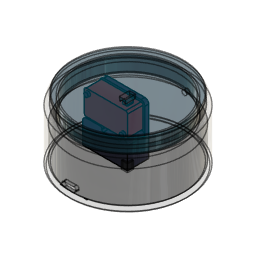
feeder (Autodesk Fusion 360 design; units mm, degrees)
part number: 2025-06-02-16-29-52-871
Autodesk Fusion 360 part; units mm, degrees
note: some values were not read from the file. Chosen so that the rebuilt part matches the saved one: which bodies a step acts on. Set by a fixed rule: which sketch regions a step uses.
sketch "Esquisse1" plane through (0, 0, 0) normal (0, 0, 1) x (1, 0, 0)
  circle A0 centre (0, 0) radius 35.5
  dimension "d1" = 71
  constraint coincident A0.centre origin
  measures "d1" diameter of A0
extrude "Extrusion1" add sketch "Esquisse1" along normal blind 2 makes body 1
sketch "Esquisse3" plane through (0, 0, 0) normal (0, 1, 0) x (1, 0, 0)
  line L0 (38.5, -1) -> (38.5, 38)
  line L1 (37.5, 39) -> (0, 39)
  line L2 (0, 39) -> (0, 37)
  line L3 (0, 37) -> (33, 37)
  line L4 (33, 37) -> (35.5, 37)
  line L5 (36.5, 36) -> (36.5, 8)
  arc A0 (36.5, 36) -> (35.5, 37) centre (35.5, 36) ccw
  arc A1 (38.5, 38) -> (37.5, 39) centre (37.5, 38) ccw
  line L6 (36, -1) -> (38.5, -1)
  line L7 (36, -1) -> (36, 4.6069)
  line L8 (36, 4.6069) -> (33, 4.6069)
  line L9 (33, 4.6069) -> (33, 12.1069)
  line L10 (33, 12.1069) -> (36.5, 15.6069)
  line L11 (33, 12.1069) -> (37.9497, 12.1069) construction
  point P0 (36.5, 37)
  dimension "d19" = 2
  dimension "d20" = 3.5
  dimension "d21" = 1
  dimension "d120" = 7.5
  dimension "d121" = 45
  constraint perpendicular L0 L1
  constraint perpendicular L1 L2
  constraint perpendicular L0 L4
  constraint perpendicular L4 L5
  constraint coincident P0 L4
  constraint coincident P0 L5
  constraint tangent L4 A0
  constraint tangent L5 A0
  constraint tangent L1 A1
  constraint tangent L0 A1
  constraint equal A0 A1
  constraint perpendicular L0 L6
  constraint horizontal L6
  constraint perpendicular L7 L8
  constraint perpendicular L8 L9
  constraint horizontal L11
  constraint coincident L5 L10.end
  measures "d19" distance of L1.end L2.end
  measures "d20" distance of L3.end P0
  measures "d21" radius of A0
  measures "d120" distance of L8.end L9.end
  measures "d121" angle of L10 L11
revolve "Révolution2" add sketch "Esquisse3" angle 360 about axis through (0, 0, 1.75) along (0, 0, 1) separate body makes body 2
sketch "Esquisse5" plane through (0, 0, 0) normal (0, 0, 1) x (1, 0, 0)
  line L0 (75, 0) -> (103, 0)
  line L1 (103, 0) -> (103, -16)
  line L2 (103, -16) -> (75, -16)
  line L3 (75, -16) -> (75, 0)
  dimension "d23" = 28
  dimension "d24" = 16
  constraint horizontal L0
  constraint vertical L1
  constraint horizontal L2
  constraint vertical L3
  measures "d23" distance of L0.start L0.end
  measures "d24" distance of L0.start L2.end
extrude "Extrusion4" add sketch "Esquisse5" along normal blind 10 separate body makes body 3
sketch "Esquisse6" plane through (0, 0, 0) normal (0, 1, 0) x (-1, 0, 0)
  line L0 (-103, 0) -> (-75, 0)
  line L1 (-75, 0) -> (-75, 10)
  line L2 (-75, 10) -> (-103, 10)
  line L3 (-103, 10) -> (-103, 0)
  line L4 (-89, 0) -> (-89, 10)
  line L5 (-75, 5) -> (-103, 5)
  line L6 (-103, 5) -> (-99.8, 5)
  line L7 (-99.8, 5) -> (-96.8, 5)
  line L8 (-98.3, 5) -> (-98.3, 3)
  line L9 (-96.8, 3) -> (-99.8, 3)
  line L10 (-99.8, 3) -> (-99.8, 7)
  line L11 (-99.8, 7) -> (-96.8, 7)
  line L12 (-96.8, 7) -> (-96.8, 3)
  dimension "d27" = 3.2
  dimension "d28" = 3
  dimension "d29" = 2
  dimension "d30" = 3
  dimension "d31" = 4
  constraint midpoint L0 L4.start
  constraint midpoint L2 L4.end
  constraint midpoint L1 L5.start
  constraint midpoint L3 L5.end
  constraint perpendicular L3 L6
  constraint perpendicular L3 L7
  constraint midpoint L7 L8.start
  constraint perpendicular L5 L8
  constraint horizontal L9
  constraint vertical L10
  constraint horizontal L11
  constraint vertical L12
  measures "d27" distance of L5.end L6.end
  measures "d28" distance of L6.end L7.end
  measures "d29" distance of L8.start L8.end
  measures "d30" distance of L9.start L9.end
  measures "d31" distance of L9.start L11.end
extrude "Extrusion5" add sketch "Esquisse6" along normal blind 2.3 contours L5 L7 L10 L11 L12 | L5 L7 L8 L9 L10 | L5 L7 L8 L9 L12 bodies 3
fillet "Congé1" radius 1.5 2 edges at (99.8, 2.3, 5) (96.8, 2.3, 5) on bodies 3
fillet "Congé2" radius 1.25 4 edges at (103, 0, 5) (75, 0, 5) (103, -16, 5) (75, -16, 5) on bodies 3
sketch "Esquisse7" plane through (0, 0, 10) normal (0, 0, 1) x (-1, 0, 0)
  arc A0 (-75, 14.75) -> (-76.25, 16) centre (-76.25, 14.75) ccw
  line L0 (-76.25, 16) -> (-101.75, 16)
  arc A1 (-101.75, 16) -> (-103, 14.75) centre (-101.75, 14.75) ccw
  line L1 (-103, 14.75) -> (-103, 1.25)
  arc A2 (-103, 1.25) -> (-101.75, 0) centre (-101.75, 1.25) ccw
  line L2 (-101.75, 0) -> (-76.25, 0)
  arc A3 (-76.25, 0) -> (-75, 1.25) centre (-76.25, 1.25) ccw
  line L3 (-75, 1.25) -> (-75, 14.75)
  line L4 (-77.5, 0) -> (-77.5, 2.5)
  line L5 (-75, 2.5) -> (-77.5, 2.5)
  line L6 (-100.5, 16) -> (-100.5, 13.5)
  line L7 (-103, 13.5) -> (-100.5, 13.5)
  circle A4 centre (-77.5, 2.5) radius 1.5
  circle A5 centre (-100.5, 13.5) radius 1.5
  dimension "d38" = 2.5
  dimension "d39" = 2.5
  dimension "d40" = 2.5
  dimension "d41" = 2.5
  dimension "d42" = 3
  dimension "d43" = 3
  constraint coincident L2 L4.start
  constraint perpendicular L2 L4
  constraint coincident L3 L5.start
  constraint perpendicular L3 L5
  constraint coincident L0 L6.start
  constraint perpendicular L0 L6
  constraint coincident L1 L7.start
  constraint perpendicular L6 L7
  constraint coincident L6.end L7.end
  constraint coincident L4.end L5.end
  measures "d38" distance of L4.start L4.end
  measures "d39" distance of L5.start L4.end
  measures "d40" distance of L6.start L6.end
  measures "d41" distance of L7.start L6.end
  measures "d42" diameter of A4
  measures "d43" diameter of A5
extrude "Extrusion6" cut sketch "Esquisse7" against normal blind 16 contours L4 L5 A4 | L4 L5 A4 | L6 L7 A5 | L6 L7 A5 bodies 3
move_body "Déplacer1" bodies 3 to x (1, 0, 0) y (0, 0, 1) z (0, -1, 0) at (0, -16, 16)
move_body "Déplacer2" bodies 3 to x (1, 0, 0) y (0, 1, 0) z (0, 0, 1) at (-98.1201, 0, -20.6266)
move_body "Déplacer3" bodies 3 to x (1, 0, 0) y (0, 1, 0) z (0, 0, 1) at (-0.2, 21, 0)
sketch "Esquisse9" plane through (0, 0, 0) normal (0, 1, 0) x (1, 0, 0)
  spline S0 degree 5 poles (-1.6476, 2.6209) (-1.623, 2.5516) (-1.5708, 2.4171) (-1.4837, 2.228) (-1.3496, 2.0009) (-1.152, 1.7603) (-0.9247, 1.5648) (-0.6696, 1.4161) (-0.3912, 1.3163) (-0.0973, 1.2661) (0.202, 1.2661) (0.4959, 1.3163) (0.7744, 1.4161) (1.0294, 1.5648) (1.2568, 1.7603) (1.4544, 2.0009) (1.5884, 2.228) (1.6756, 2.4171) (1.7278, 2.5516) (1.7524, 2.6209) knots 0 0 0 0 0 0 0.066667 0.133333 0.2 0.266667 0.333333 0.4 0.466667 0.533333 0.6 0.666667 0.733333 0.8 0.866667 0.933333 1 1 1 1 1 1
  line L0 (0, 0) -> (2, 0)
  line L1 (0, 0) -> (-2, 0)
  line L2 (-2, 0) -> (-1.6476, 2.6209)
  line L3 (2, 0) -> (1.7524, 2.6209)
  point P0 (-0.6476, 1.4209)
  point P1 (0.7524, 1.4209)
  dimension "d46" = 2
  dimension "d47" = 2
  constraint coincident L0.start L1.start
  constraint horizontal L0
  constraint horizontal L1
  measures "d46" distance of L0.start L0.end
  measures "d47" distance of L0.start L1.end
extrude "Extrusion7" add sketch "Esquisse9" along normal blind 2.9 and the other way blind 3.6 bodies 1
sketch "Esquisse10" plane through (0, 0, -37) normal (0, 0, 1) x (-1, 0, 0)
  circle A0 centre (0, 0) radius 35.5
  line L0 (23.6914, 5.6619) -> (-5.3086, 5.6619)
  line L1 (-5.3086, 5.6619) -> (-5.3086, -5.6058)
  line L2 (-5.3086, -5.6058) -> (23.6914, -5.6058)
  line L3 (23.6914, -5.6058) -> (23.6914, 5.6619)
  line L4 (-5.3086, -5.6058) -> (23.6914, -5.6058)
  line L5 (23.6914, -5.6058) -> (23.6914, -8.1058)
  line L6 (23.6914, -8.1058) -> (-5.3086, -8.1058)
  line L7 (-5.3086, -8.1058) -> (-5.3086, -5.6058)
  dimension "d53" = 2.5
  dimension "d54" = 29
  dimension "d55" = 29
  constraint horizontal L0
  constraint vertical L1
  constraint horizontal L2
  constraint vertical L3
  constraint horizontal L4
  constraint vertical L5
  constraint horizontal L6
  constraint vertical L7
  measures "d53" distance of L1.end L6.end
  measures "d54" distance of L1.end L2.end
  measures "d55" distance of L5.end L6.end
extrude "Extrusion8" add sketch "Esquisse10" along normal blind 16.3 separate body contours L0 L1 L2 L3 L4 makes body 4
extrude "Extrusion9" add sketch "Esquisse10" along normal blind 33 contours L2 L4 L5 L6 L7 bodies 4
sketch "Esquisse11" plane through (0, 5.6058, 0) normal (0, -1, 0) x (1, 0, 0)
  line L0 (-23.6914, -20.7) -> (5.3086, -20.7)
  line L1 (5.3086, -20.7) -> (5.3086, -4)
  line L2 (5.3086, -4) -> (-23.6914, -4)
  line L3 (-23.6914, -4) -> (-23.6914, -20.7)
  circle A0 centre (-20.8196, -7.125) radius 1.5
  circle A1 centre (2.18, -18.125) radius 1.5
  circle A2 centre (-20.8196, -7.125) radius 1.425
  circle A3 centre (2.18, -18.125) radius 1.425
  dimension "d60" = 3
  dimension "d61" = 3
  dimension "d62" = 2.85
  dimension "d63" = 2.85
  constraint concentric A0 A2
  constraint concentric A1 A3
  measures "d60" diameter of A0
  measures "d61" diameter of A1
  measures "d62" diameter of A2
  measures "d63" diameter of A3
extrude "Extrusion10" add sketch "Esquisse11" along normal blind 12 contours A2 | A3 bodies 2 3 1 4
fillet "Congé3" radius 2.5 4 edges at (5.3086, -0.028, -20.7) (5.3086, 6.8558, -4) (-23.6914, 6.8558, -4) (-23.6914, -0.028, -20.7) on bodies 4
sketch "Esquisse15" plane through (0, -5.6619, 0) normal (0, -1, 0) x (1, 0, 0)
  arc A0 (-21.1914, -20.7) -> (-23.6914, -23.2) centre (-21.1914, -23.2) ccw
  line L0 (-23.6914, -23.2) -> (-23.6914, -37)
  line L1 (-23.6914, -37) -> (5.3086, -37)
  line L2 (5.3086, -37) -> (5.3086, -23.2)
  arc A1 (5.3086, -23.2) -> (2.8086, -20.7) centre (2.8086, -23.2) ccw
  line L3 (2.8086, -20.7) -> (-21.1914, -20.7)
  line L4 (0.9717, -23.2) -> (-11.3065, -23.2)
  line L5 (-11.3065, -23.2) -> (-11.3065, -20.7)
  line L6 (-11.3065, -20.7) -> (0.9717, -20.7)
  line L7 (0.9717, -20.7) -> (0.9717, -23.2)
  constraint horizontal L4
  constraint vertical L5
  constraint horizontal L6
  constraint vertical L7
  constraint coincident L3 L5.end
extrude "Extrusion18" cut sketch "Esquisse15" against normal blind 31 contours L3 L4 L5 L6 L7 bodies 4
fillet "Congé6" radius 1 2 edges at (-11.3065, -0.028, -20.7) (0.9717, -0.028, -20.7) on bodies 4
fillet "Congé7" radius 1 2 edges at (0.9717, 1.222, -23.2) (-11.3065, 1.222, -23.2) on bodies 4
sketch "Esquisse16" plane through (0, 0, 0) normal (0, 0, -1) x (1, 0, 0)
  line L0 (-2, 3.6) -> (2, 3.6)
  line L1 (2, 3.6) -> (2, -2.9)
  line L2 (2, -2.9) -> (-2, -2.9)
  line L3 (-2, -2.9) -> (-2, 3.6)
  circle A0 centre (0, 0) radius 35.5
  circle A1 centre (0, 0) radius 32.9
  circle A2 centre (0, 0) radius 31.9
  dimension "d118" = 65.8
  dimension "d119" = 63.8
  constraint coincident A0.centre A1.centre
  measures "d118" diameter of A1
  measures "d119" diameter of A2
extrude "Extrusion19" add sketch "Esquisse16" along normal blind 10 contours A1 bodies 1
sketch "Esquisse12" plane through (0, 0, -37) normal (0, 0, 1) x (-1, 0, 0)
  line L0 (-5.31, 5.66) -> (-5.3919, 5.7174)
  line L1 (-5.31, 5.66) -> (-5.21, 5.66) construction
  line L2 (-5.3919, 5.7174) -> (-2.3919, 5.7174)
  line L3 (-2.3919, 5.7174) -> (-2.3919, 6.7174)
  line L4 (-2.3919, 6.7174) -> (-5.3919, 6.7174)
  line L5 (-5.3919, 6.7174) -> (-5.3919, 5.7174)
  line L6 (-5.3919, 5.7174) -> (-6.3919, 5.7174)
  line L7 (-6.3919, 5.7174) -> (-6.3919, 2.7174)
  line L8 (-6.3919, 2.7174) -> (-5.3919, 2.7174)
  line L9 (-5.3919, 2.7174) -> (-5.3919, 5.7174)
  line L10 (23.6913, -8.1056) -> (23.7621, -8.1763)
  line L11 (23.6913, -8.1056) -> (23.7913, -8.1056) construction
  line L12 (23.7621, -8.1763) -> (24.7621, -8.1763)
  line L13 (24.7621, -8.1763) -> (24.7621, -5.1763)
  line L14 (24.7621, -5.1763) -> (23.7621, -5.1763)
  line L15 (23.7621, -5.1763) -> (23.7621, -8.1763)
  line L16 (23.7621, -8.1763) -> (20.7621, -8.1763)
  line L17 (20.7621, -8.1763) -> (20.7621, -9.1763)
  line L18 (20.7621, -9.1763) -> (23.7621, -9.1763)
  line L19 (23.7621, -9.1763) -> (23.7621, -8.1763)
  dimension "d68" = 145
  dimension "d69" = 0.1
  dimension "d70" = 3
  dimension "d71" = 1
  dimension "d72" = 1
  dimension "d73" = 3
  dimension "d74" = 45
  dimension "d75" = 0.1
  dimension "d76" = 1
  dimension "d77" = 3
  dimension "d78" = 3
  dimension "d79" = 1
  constraint horizontal L1
  constraint horizontal L2
  constraint vertical L3
  constraint horizontal L4
  constraint vertical L5
  constraint horizontal L6
  constraint vertical L7
  constraint horizontal L8
  constraint vertical L9
  constraint horizontal L11
  constraint horizontal L12
  constraint vertical L13
  constraint horizontal L14
  constraint vertical L15
  constraint horizontal L16
  constraint vertical L17
  constraint horizontal L18
  constraint vertical L19
  measures "d68" angle of L0 L1
  measures "d69" distance of L0.start L0.end
  measures "d70" distance of L0.end L2.end
  measures "d71" distance of L0.end L4.end
  measures "d72" distance of L0.end L6.end
  measures "d73" distance of L0.end L8.end
  measures "d74" angle of L10 L11
  measures "d75" distance of L10.start L10.end
  measures "d76" distance of L10.end L12.end
  measures "d77" distance of L10.end L14.end
  measures "d78" distance of L10.end L16.end
  measures "d79" distance of L10.end L18.end
extrude "Extrusion11" add sketch "Esquisse12" along normal blind 5 separate body makes body 6 at (-22.7621, 8.1763, -35.3333) makes body 6 at (-23.7621, 6.1763, -35.3333) makes body 7 at (5.3919, -3.7174, -35.3333) makes body 7 at (3.3919, -6.7174, -35.3333)
extrude "Extrusion12" add 1 faces at (5.3919, -6.384, -35.3333) along direction (1, 0, 0) blind 1 on bodies 7 bodies 2 4 6 7
extrude "Extrusion13" add 1 faces at (-23.7621, 8.843, -35.3333) along direction (-1, 0, 0) blind 1 on bodies 6 bodies 2 4 6
sketch "Esquisse13" plane through (0, 0, 0) normal (0, 0, 1) x (1, 0, 0)
  line L0 (69, 2) -> (86.5, 2)
  line L1 (86.5, 2) -> (86.5, -26)
  line L2 (86.5, -26) -> (69, -26)
  line L3 (69, -26) -> (69, 2)
  line L4 (77.75, 2) -> (77.75, -26)
  line L5 (77.75, -26) -> (82.35, -26)
  line L6 (82.35, -26) -> (82.35, -27.5)
  line L7 (82.35, -27.5) -> (77.75, -27.5)
  line L8 (77.75, -27.5) -> (77.75, -26)
  line L9 (77.75, -26) -> (73.15, -26)
  line L10 (73.15, -26) -> (73.15, -27.5)
  line L11 (73.15, -27.5) -> (77.75, -27.5)
  line L12 (77.75, -27.5) -> (77.75, -26)
  line L13 (73.15, -27.5) -> (82.35, -27.5)
  line L14 (82.35, -27.5) -> (82.35, -20)
  line L15 (82.35, -20) -> (73.15, -20)
  line L16 (73.15, -20) -> (73.15, -27.5)
  dimension "d86" = 17.5
  dimension "d87" = 28
  dimension "d88" = 4.6
  dimension "d89" = 1.5
  dimension "d90" = 4.6
  dimension "d91" = 9.2
  dimension "d92" = 7.5
  constraint horizontal L0
  constraint vertical L1
  constraint horizontal L2
  constraint vertical L3
  constraint midpoint L0 L4.start
  constraint midpoint L2 L4.end
  constraint horizontal L5
  constraint vertical L6
  constraint horizontal L7
  constraint vertical L8
  constraint horizontal L9
  constraint vertical L10
  constraint horizontal L11
  constraint vertical L12
  constraint horizontal L13
  constraint vertical L14
  constraint horizontal L15
  constraint vertical L16
  measures "d86" distance of L0.start L0.end
  measures "d87" distance of L0.start L2.end
  measures "d88" distance of L4.end L5.end
  measures "d89" distance of L4.end L7.end
  measures "d90" distance of L4.end L9.end
  measures "d91" distance of L10.end L6.end
  measures "d92" distance of L10.end L15.end
extrude "Extrusion14" add sketch "Esquisse13" along normal blind 3 separate body contours L0 L2 L3 L4 L15 L16 | L0 L1 L2 L4 L14 L15 | L2 L4 L5 L14 L15 | L2 L4 L9 L15 L16 makes body 8
extrude "Extrusion15" add sketch "Esquisse13" along normal blind 6.2 and the other way blind -3 contours L2 L4 L5 L14 L15 | L2 L4 L9 L15 L16 | L2 L8 L9 L10 L11 L12 L13 L16 | L2 L5 L6 L7 L8 L12 L13 L14 bodies 8
extrude "Extrusion16" add 1 faces at (79.2833, -27.5, 4.0667) along direction (0, -1, 0) blind 4 on bodies 8 bodies 8
fillet "Congé4" radius 1.5 4 edges at (82.35, -23.75, 6.2) (73.15, -23.75, 6.2) (73.15, -26.75, 3) (82.35, -26.75, 3) on bodies 8
move_body "Déplacer4" bodies 8 to x (1, 0, 0) y (0, 1, 0) z (0, 0, 1) at (-77.7607, -9.1, -36.9765)
copy_body "Copier/Coller des corps1" bodies 8 makes body 9
move_body "Déplacer5" bodies 9 to x (1, 0, 0) y (0, 1, 0) z (0, 0, 1) at (0, -34, 0)
combine "Combiner1" operation cut target body 2 tool bodies 8
move_body "Déplacer6" bodies 9 to x (1, 0, 0) y (0, 1, 0) z (0, 0, 1) at (0, 34, 0)
sketch "Esquisse14" plane through (0, 0, 0) normal (0, 1, 0) x (1, 0, 0)
  circle A0 centre (0, 17) radius 1.55
  dimension "d103" = 3.1
  measures "d103" diameter of A0
extrude "Extrusion17" cut sketch "Esquisse14" along normal blind 83 and the other way blind -31 bodies 2
fillet "Congé5" radius 10.5 1 edges at (-35.8946, -13.9222, 1) on bodies 2
hidden bodies 9
equation "d20 = 5.5 mm - 2 mm"
equation "d95 = 3 mm + 3.2 mm"
named bodies: "top", "base", "latch_switch", "latch_support", "chargeur", "chargeur (1)"
